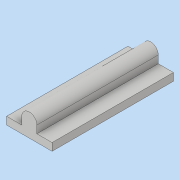
# Autodesk Inventor part: lw_5_корпус
Saved by Autodesk Inventor 2019 (Build 230136000, 136)
## iProperties
Created: 2021-04-29
Part Number: lw_5_корпус
Material: Типовые
Document SubType Name: Modeling
Designer: Kurbatova
Density: 1 g/cm^3
Appearance: По умолчанию
Author: Kurbatova
Autodesk Inventor part; units mm, degrees
ref_plane "YZ Plane" through (0, 0, 0) normal (1, 0, 0) x (0, 1, 0)
ref_plane "XZ Plane" through (0, 0, 0) normal (0, 1, 0) x (-1, 0, 0)
ref_plane "XY Plane" through (0, 0, 0) normal (0, 0, 1) x (1, 0, 0)
sketch "Эскиз8" plane through (0, 0, 0) normal (0, 0, 1) x (1, 0, 0)
  line L0 (0, 5) -> (0, -5)
  line L1 (-5, 0) -> (5, 0)
  arc A0 (5, 0) -> (-5, 0) centre (0, 0) ccw
  line L2 (-5, 0) -> (-5, -5)
  line L3 (5, 0) -> (5, -5)
  line L4 (0, -5) -> (-4, -5)
  line L5 (4, -5) -> (0, -5)
  line L6 (-4, -5) -> (-4, 0)
  arc A1 (4, 0) -> (-4, 0) centre (0, 0) ccw
  line L7 (4, 0) -> (4, -5)
  line L8 (-5, -5) -> (-4, -5)
  line L9 (4, -5) -> (5, -5)
  line L10 (-15, -5) -> (-5, -5)
  line L11 (0, -5) -> (-5, -5)
  line L12 (5, -5) -> (0, -5)
  line L13 (5, -5) -> (15, -5)
  line L14 (-15, -10) -> (15, -10)
  line L15 (-15, -5) -> (-15, -10)
  line L16 (-15, -5) -> (15, -5)
  line L17 (15, -10) -> (15, -5)
  line L18 (15, -10) -> (-15, -10)
  line L19 (-15, -5) -> (-15, -10)
  dimension "d32" = 10
  dimension "d33" = 5
  dimension "d34" = 5
  dimension "d52" = 1
  constraints: 40 end point, 5 point on circle, 4 collinear, 3 horizontal, 3 vertical, 2 centre point, 2 midpoint, 2 tangent, 1 coincident, 1 perpendicular, 2 other
  measures "d32" diameter of A0
  measures "d33" distance of L1.start L2.end
  measures "d34" distance of L1.end L3.end
  measures "d52" radial gap between concentric circles of A0 A1
sketch "Эскиз9" plane through (0, 0, 0) normal (0, 0, 1) x (1, 0, 0)
  line L0 (-15, -5) -> (-5, -5)
  line L1 (0, -5) -> (-5, -5)
  line L2 (5, -5) -> (0, -5)
  line L3 (5, -5) -> (15, -5)
  line L4 (-15, -10) -> (15, -10)
  line L5 (-15, -5) -> (-15, -10)
  line L6 (-15, -5) -> (15, -5)
  line L7 (15, -10) -> (15, -5)
  line L8 (15, -10) -> (-15, -10)
  line L9 (-15, -5) -> (-15, -10)
  constraints: 20 end point, 3 collinear, 1 perpendicular
extrude "Выдавливание9" [suppressed]
extrude "Выдавливание14" add sketch "Эскиз8" along normal blind 80
sketch "Эскиз10" plane through (-5, -5, 0) normal (-1, 0, 0) x (0, 0, 1)
  line L0 (0, 10) -> (80, 10) projected
  line L1 (0, 0) -> (80, 0) projected
  line L2 (0, 5) -> (80, 5) projected
  line L3 (7.9097, 10) -> (7.9097, 0)
  line L4 (0, 0) -> (80, 0) projected
  line L5 (11.9885, 0) -> (11.9885, 5)
  line L6 (7.9097, 0) -> (11.9885, 0)
  line L7 (11.9885, 5) -> (23.7841, 5)
  line L8 (23.7841, 0) -> (11.9885, 0)
  line L9 (23.7841, 5) -> (23.7841, 0)
  line L10 (7.9097, 10) -> (28.0834, 10)
  line L11 (28.0834, 0) -> (28.0834, 10)
  line L12 (28.0834, 0) -> (23.7841, 0)
  constraints: 18 end point, 8 point on line, 4 perpendicular, 2 collinear, 1 vertical
extrude "Выдавливание15" cut sketch "Эскиз10" against normal blind 2 contours L0 L11 L2 L3 | L2 L5 L1 L3 | L11 L1 L9 L2
shell "Оболочка3" thickness 1 removed faces 1 at (-3, 2.6667, 19.9257)
equation "\"d32\" = diametr_"
equation "\"diametr_\" = 10"
